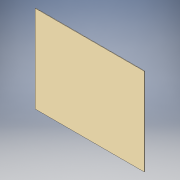
# Autodesk Inventor part: gatorboard_01875in
Saved by Autodesk Inventor 2019 (Build 230136000, 136)
## iProperties
Created: 2019-03-10
Part Number: gatorboard_01875in
Material: Generic
Document SubType Name: Modeling
Designer: Wilson Lab
Density: 1 g/cm^3
Appearance: Default
Author: Wilson Lab
Autodesk Inventor part; units mm, degrees
ref_plane "YZ Plane" through (0, 0, 0) normal (1, 0, 0) x (0, 1, 0)
ref_plane "XZ Plane" through (0, 0, 0) normal (0, 1, 0) x (-1, 0, 0)
ref_plane "XY Plane" through (0, 0, 0) normal (0, 0, 1) x (1, 0, 0)
sketch "Sketch1" plane through (0, 0, 0) normal (0, 0, 1) x (1, 0, 0)
  line L0 (0, 0) -> (1016, 0)
  line L1 (1016, 0) -> (1016, 812.8)
  line L2 (1016, 812.8) -> (0, 812.8)
  line L3 (0, 812.8) -> (0, 0)
  dimension "d2" = 1016
  dimension "d3" = 812.8
  constraints: 8 end point, 2 parallel, 1 coincident, 1 horizontal, 1 perpendicular
  measures "d2" distance of L1.end L2.end
  measures "d3" distance of L0.end L1.end
extrude "Extrusion1" add sketch "Sketch1" along normal blind 4.7625
body "Solid1"
